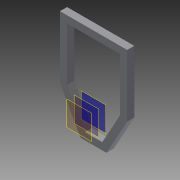
# Autodesk Inventor part: alignment_tool
Saved by Autodesk Inventor 2015 SP1 (Build 190203100, 203)
## iProperties
Created: 2015-09-17
Part Number: alignment_tool
Material: Generic
Document SubType Name: Modeling
Designer: tankadmin
Density: 1 g/cm^3
Appearance: Default
Author: tankadmin
Autodesk Inventor part; units mm, degrees
ref_plane "YZ Plane" through (0, 0, 0) normal (1, 0, 0) x (0, 1, 0)
ref_plane "XZ Plane" through (0, 0, 0) normal (0, 1, 0) x (-1, 0, 0)
ref_plane "XY Plane" through (0, 0, 0) normal (0, 0, 1) x (1, 0, 0)
sketch "Sketch1" plane through (0, 0, 0) normal (0, 0, 1) x (1, 0, 0)
  line L0 (-44.45, -76.2) -> (44.45, -76.2)
  line L1 (44.45, -76.2) -> (44.45, -19.05)
  line L2 (44.45, -19.05) -> (22.614, -6.964)
  line L3 (22.614, -6.964) -> (37.9893, 20.8148)
  line L4 (37.9893, 20.8148) -> (75.5958, 0)
  line L5 (75.5958, 0) -> (139.7, 0)
  line L6 (139.7, 0) -> (139.7, 76.2)
  line L7 (139.7, 76.2) -> (-139.7, 76.2)
  line L8 (-139.7, 76.2) -> (-139.7, 0)
  line L9 (-139.7, 0) -> (-75.5958, 0)
  line L10 (-75.5958, 0) -> (-37.9893, 20.8148)
  line L11 (-37.9893, 20.8148) -> (-22.614, -6.964)
  line L12 (-22.614, -6.964) -> (-44.45, -19.05)
  line L13 (-44.45, -19.05) -> (-44.45, -76.2)
  line L14 (0, -76.2) -> (0, 76.2) construction
  line L15 (-127, 63.5) -> (127, 63.5)
  line L16 (127, 63.5) -> (127, 12.7)
  line L17 (127, 12.7) -> (73.6309, 12.7)
  line L18 (73.6309, 12.7) -> (34.0201, 34.6241)
  line L19 (34.0201, 34.6241) -> (8.8047, -10.9331)
  line L20 (8.8047, -10.9331) -> (31.75, -23.6331)
  line L21 (31.75, -23.6331) -> (31.75, -63.5)
  line L22 (31.75, -63.5) -> (-31.75, -63.5)
  line L23 (-31.75, -63.5) -> (-31.75, -23.6331)
  line L24 (-31.75, -23.6331) -> (-8.8047, -10.9331)
  line L25 (-8.8047, -10.9331) -> (-34.0201, 34.6241)
  line L26 (-34.0201, 34.6241) -> (-73.6309, 12.7)
  line L27 (-73.6309, 12.7) -> (-127, 12.7)
  line L28 (-127, 12.7) -> (-127, 63.5)
  line L29 (139.7, 38.1) -> (-139.7, 38.1) construction
  line L30 (139.7, 19.05) -> (-139.7, 19.05) construction
  point P0 (0, 0)
  point P1 (0, 0)
  point P2 (0, 19.05)
  point P3 (25.4, 19.05)
  point P4 (-25.4, 19.05)
  dimension "d2" = 88.9
  dimension "d3" = 57.15
  dimension "d4" = 279.4
  dimension "d5" = 152.4
  dimension "d8" = 76.2
  dimension "d10" = 12.7
  dimension "d11" = 10.16
  dimension "d12" = 10.16
  dimension "d13" = 10.16
  dimension "d14" = 12.7
  dimension "d15" = 10.16
  dimension "d16" = 10.16
  dimension "d17" = 10.16
  dimension "d18" = 12.7
  dimension "d19" = 12.7
  dimension "d96" = 114.3
  dimension "d97" = 19.05
  dimension "d98" = 25.4
  dimension "d99" = 31.75
  dimension "d100" = 25.4
  dimension "d101" = 31.75
  dimension "d102" = 12.7
  constraints: 62 end point, 17 perpendicular, 8 point on line, 6 midpoint, 2 equal length, 1 coincident, 1 horizontal, 4 other
  measures "d2" distance between parallel lines of L1 L13
  measures "d3" distance of L0.end L1.end
  measures "d4" distance between parallel lines of L6 L8
  measures "d5" distance between parallel lines of L0 L7
  measures "d8" distance between parallel lines of L0 L9
  measures "d10" distance between parallel lines of L22 L0
  measures "d11" distance between parallel lines of L24 L12
  measures "d12" distance between parallel lines of L25 L11
  measures "d13" distance between parallel lines of L10 L26
  measures "d14" distance between parallel lines of L9 L27
  measures "d15" distance between parallel lines of L2 L20
  measures "d16" distance between parallel lines of L3 L19
  measures "d17" distance between parallel lines of L4 L18
  measures "d18" distance between parallel lines of L5 L17
  measures "d19" distance between parallel lines of L6 L16
  measures "d96" distance between parallel lines of L0 L29
  measures "d97" distance between parallel lines of L30 L29
  measures "d98" distance of point (0, 19.05) point (25.4, 19.05)
  measures "d99" distance between parallel lines of L2 L4
  measures "d100" distance of point (-25.4, 19.05) point (0, 19.05)
  measures "d101" distance between parallel lines of L10 L12
  measures "d102" vertical distance of L19.end L20.end
ref_plane "Work Plane2" through (0, 0, 6.35) normal (0, 0, 1) x (1, 0, 0)
ref_plane "Work Plane4" through (0, 0, 12.7) normal (0, 0, 1) x (1, 0, 0)
ref_plane "Work Plane3" through (0, 0, 6.35) normal (0, 0, -1) x (-1, 0, 0)
ref_plane "Work Plane1" through (0, 0, 0) normal (0, 0, -1) x (-1, 0, 0)
ref_plane "Work Plane6" through (0, 0, 0) normal (0, 0, -1) x (-1, 0, 0)
sketch "Sketch7" plane through (0, 0, 0) normal (0, 0, -1) x (-1, 0, 0)
  line L0 (-8.8047, -10.9331) -> (-34.0201, 34.6241) construction
  line L1 (-31.75, -23.6331) -> (-8.8047, -10.9331) construction
  line L2 (-34.0201, 34.6241) -> (-73.6309, 12.7) projected
  line L3 (35.56, 63.5) -> (25.4, 63.5)
  line L4 (25.4, 63.5) -> (25.4, 19.05)
  line L5 (35.56, 33.7718) -> (35.56, 63.5)
  line L6 (127, 63.5) -> (-127, 63.5) construction
  line L7 (0, -76.2) -> (0, 76.2) construction
  line L8 (-35.56, 33.7718) -> (-35.56, 63.5)
  line L9 (-35.56, 63.5) -> (-25.4, 63.5)
  line L10 (-25.4, 63.5) -> (-25.4, 19.05)
  line L11 (-25.4, 19.05) -> (-35.56, 33.7718)
  line L12 (-139.7, 19.05) -> (139.7, 19.05) construction
  line L13 (35.56, 33.7718) -> (25.4, 19.05)
  line L14 (34.0201, 34.6241) -> (73.6309, 12.7) construction
  point P0 (0, 0)
  dimension "d120" = 25.4
  dimension "d121" = 10.16
  constraints: 16 end point, 4 symmetric about line, 2 point on line, 1 collinear
  measures "d120" distance between parallel lines of L7 L4
  measures "d121" distance between parallel lines of L5 L4
ref_plane "Work Plane5" through (0, 0, 0) normal (0, 0, -1) x (-1, 0, 0)
sketch "Sketch8" plane through (0, 0, 0) normal (0, 0, -1) x (-1, 0, 0)
  line L0 (-30.48, 63.5) -> (-30.48, 7.5779)
  line L1 (-30.48, 7.5779) -> (-11.7992, -26.1731)
  line L2 (-11.7992, -26.1731) -> (11.7992, -26.1731)
  line L3 (11.7992, -26.1731) -> (30.48, 7.5779)
  line L4 (30.48, 7.5779) -> (30.48, 63.5)
  line L5 (30.48, 63.5) -> (-30.48, 63.5)
  line L6 (-25.4, 63.5) -> (25.4, 63.5) construction
  line L7 (-23.622, 56.642) -> (-23.622, 9.3492)
  line L8 (-23.622, 9.3492) -> (-7.7566, -19.3151)
  line L9 (-7.7566, -19.3151) -> (7.7566, -19.3151)
  line L10 (7.7566, -19.3151) -> (23.622, 9.3492)
  line L11 (23.622, 9.3492) -> (23.622, 56.642)
  line L12 (23.622, 56.642) -> (-23.622, 56.642)
  line L13 (-29.972, 62.992) -> (-29.972, 7.7091)
  line L14 (-29.972, 7.7091) -> (-11.4997, -25.6651)
  line L15 (-11.4997, -25.6651) -> (11.4997, -25.6651)
  line L16 (11.4997, -25.6651) -> (29.972, 7.7091)
  line L17 (29.972, 7.7091) -> (29.972, 62.992)
  line L18 (29.972, 62.992) -> (-29.972, 62.992)
  point P0 (0, 0)
  dimension "d111" = 0
  dimension "d126" = 60.96
  dimension "d127" = 6.35
  dimension "d128" = 0.508
  dimension "d131" = 151.036
  dimension "d134" = 63.5
  dimension "d135" = 30.48
  dimension "d136" = 55.9221
  dimension "d137" = 33.751
  constraints: 38 end point, 6 perpendicular, 3 parallel, 2 equal length, 1 vertical, 10 other
  measures "d111" distance between parallel lines of L6 L5
  measures "d126" distance between parallel lines of L0 L4
  measures "d127" distance between parallel lines of L13 L7
  measures "d128" distance between parallel lines of L0 L13
  measures "d131" angle of L4 L3
  measures "d134" distance from line of point (0, 0) L5
  measures "d135" distance from line of point (0, 0) L0
  measures "d136" distance of L3.end L4.end
  measures "d137" vertical distance of L2.end L3.end
extrude "Extrusion14" add sketch "Sketch8" along normal blind 6.35 contours L18 L17 L16 L15 L14 L13
equation "\"d11\" = d13"
equation "\"d12\" = d13"
equation "\"d14\" = d10"
equation "\"d15\" = d13"
equation "\"d16\" = d13"
equation "\"d17\" = d13"
equation "\"d18\" = d10"
equation "\"d19\" = d10"
body "Solid2"
